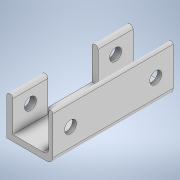
# Autodesk Inventor part: CableChain_Holder
Saved by Autodesk Inventor 2021 (Build 250183000, 183)
## iProperties
Created: 2021-12-04
Part Number: CableChain_Holder
Material: Generic
Document SubType Name: Modeling
Designer: Jorian Brusind
Density: 1 g/cm^3
Appearance: Default
Author: Jorian Brusind
Autodesk Inventor part; units mm, degrees
ref_plane "YZ Plane" through (0, 0, 0) normal (1, 0, 0) x (0, 1, 0)
ref_plane "XZ Plane" through (0, 0, 0) normal (0, 1, 0) x (-1, 0, 0)
ref_plane "XY Plane" through (0, 0, 0) normal (0, 0, 1) x (1, 0, 0)
sketch "Sketch1" plane through (0, 0, 0) normal (0, 1, 0) x (-1, 0, 0)
  line L0 (0, 0) -> (23, 0)
  line L1 (23, 0) -> (23, -60)
  line L2 (23, -60) -> (0, -60)
  line L3 (0, -60) -> (0, 0)
  dimension "d0" = 23
  dimension "d1" = 60
  constraints: 8 end point, 2 parallel, 1 horizontal, 1 perpendicular
  measures "d0" distance of L1.end L2.end
  measures "d1" distance of L0.end L1.end
extrude "Extrusion1" add sketch "Sketch1" along normal blind 3
sketch "Sketch2" plane through (0, 3, 0) normal (0, 1, 0) x (1, 0, 0)
  line L0 (-23, 0) -> (0, 0) projected
  line L1 (0, 0) -> (-2, 0)
  line L2 (-2, 0) -> (-2, 60)
  line L3 (-2, 60) -> (0, 60)
  line L4 (0, 60) -> (0, 0)
  dimension "d4" = 2
  dimension "d5" = 60
  constraints: 8 end point, 2 parallel, 1 horizontal, 1 perpendicular
  measures "d4" distance of L2.end L3.end
  measures "d5" distance of L1.end L2.end
extrude "Extrusion2" add sketch "Sketch2" along normal blind 20
sketch "Sketch3" plane through (0, 0, 0) normal (0, -1, 0) x (1, 0, 0)
  line L0 (-23, 0) -> (0, 0) projected
  line L1 (0, -60) -> (-23, -60) projected
  line L2 (-23, 0) -> (-20, 0)
  line L3 (-20, 0) -> (-20, -60)
  line L4 (-20, -60) -> (-23, -60)
  line L5 (-23, -60) -> (-23, 0)
  point P0 (-20, 0)
  dimension "d8" = 3
  constraints: 8 end point, 2 parallel, 1 horizontal, 1 perpendicular, 1 point on line
  measures "d8" distance of L3.end L4.end
extrude "Extrusion3" add sketch "Sketch3" against normal blind 20
sketch "Sketch4" plane through (-20, 0, 0) normal (1, 0, 0) x (0, 0, 1)
  line L0 (0, 0) -> (0, -20) projected
  line L1 (0, -8.5) -> (10, -8.5)
  line L2 (-60, -3) -> (-60, -20) projected
  circle A0 centre (10, -8.5) radius 3
  line L3 (0, -20) -> (-60, -20) projected
  line L4 (0, -20) -> (-60, -20)
  circle A1 centre (50, -8.5) radius 3
  point P0 (0, 3)
  point P1 (60, 0)
  dimension "d11" = 10
  dimension "d12" = 6
  dimension "d15" = 40
  constraints: 4 end point, 2 centre point, 2 horizontal, 1 coincident, 1 collinear, 1 point on line, 3 other
  measures "d11" distance of L1.start L1.end
  measures "d12" diameter of A0
  measures "d15" distance of A0.centre A1.centre
extrude "Extrusion4" cut sketch "Sketch4" against normal through all
fillet "Fillet3" radius 3 2 edges at (-2, 3, -30) (0, 0, -30)
fillet "Fillet4" radius 1 2 edges at (0, 23, -30) (-2, 23, -30)
sketch "Sketch6" plane through (-23, 0, -60) normal (-1, 0, 0) x (0, 0, 1)
  line L0 (0, 3) -> (60, 3) projected
  line L1 (30, 3) -> (30, 10)
  line L2 (30, 3) -> (42.5, 3)
  line L3 (42.5, 3) -> (17.5, 3)
  line L4 (17.5, 3) -> (17.5, 20)
  line L5 (17.5, 20) -> (42.5, 20)
  line L6 (42.5, 20) -> (42.5, 3)
  point P0 (60, 0)
  dimension "d32" = 7
  dimension "d33" = 12.5
  dimension "d34" = 25
  dimension "d35" = 17
  constraints: 12 end point, 2 parallel, 1 horizontal, 1 midpoint, 1 perpendicular, 1 point on line, 1 vertical
  measures "d32" distance of L1.start L1.end
  measures "d33" distance of L1.start L2.end
  measures "d34" distance of L4.end L5.end
  measures "d35" distance of L3.end L4.end
extrude "Extrusion6" cut sketch "Sketch6" against normal blind 6
sketch "Sketch7" plane through (-23, 0, -60) normal (-1, 0, 0) x (0, 0, 1)
  line L0 (42.5, 17) -> (60, 17) projected
  line L1 (51.25, 17) -> (51.25, 12)
  line L2 (0, 0) -> (60, 0) projected
  circle A0 centre (51.25, 12) radius 3
  line L3 (17.5, 17) -> (0, 17) projected
  line L4 (0, 22) -> (60, 22) projected
  line L5 (8.75, 17) -> (8.75, 0)
  line L6 (60, 0) -> (0, 0) projected
  line L7 (51.25, 12) -> (8.75, 12)
  circle A1 centre (8.75, 12) radius 3
  dimension "d38" = 5
  dimension "d39" = 6
  dimension "d41" = 6
  constraints: 6 end point, 3 perpendicular, 2 centre point, 2 coincident, 2 midpoint, 2 point on line, 1 other
  measures "d38" distance of L1.start L1.end
  measures "d39" diameter of A0
  measures "d41" diameter of A1
extrude "Extrusion7" cut sketch "Sketch7" against normal through all
fillet "Fillet6" radius 1.5 4 edges at (-23, 20, -8.75) (-20, 20, -8.75) (-23, 20, -51.25) (-20, 20, -51.25)
body "Solid1"
